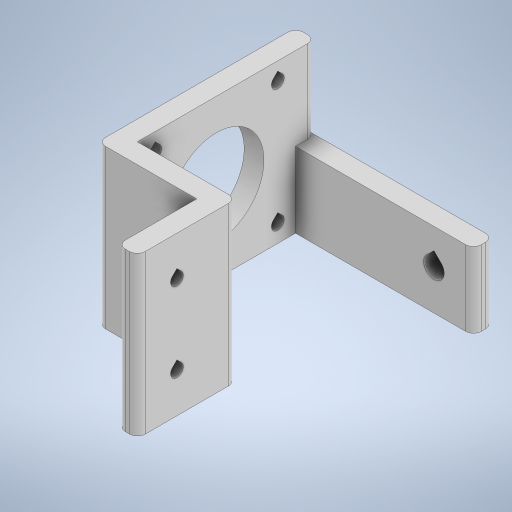
# Autodesk Inventor part: Motor Mount Redesign
Saved by Autodesk Inventor 2023.1 (Build 271208000, 208)
## iProperties
Created: 2022-11-21
Part Number: Motor Mount Redesign
Material: Generic
Document SubType Name: Modeling
Designer: nicol
Density: 1 g/cm^3
Appearance: Default
Author: nicol
Autodesk Inventor part; units mm, degrees
ref_plane "YZ Plane" through (0, 0, 0) normal (1, 0, 0) x (0, 1, 0)
ref_plane "XZ Plane" through (0, 0, 0) normal (0, 1, 0) x (-1, 0, 0)
ref_plane "XY Plane" through (0, 0, 0) normal (0, 0, 1) x (1, 0, 0)
sketch "Sketch1" plane through (0, 0, 0) normal (0, 1, 0) x (-1, 0, 0)
  line L0 (0, 0) -> (0, -25)
  line L1 (0, -25) -> (25, -25)
  line L2 (25, -25) -> (25, -65)
  line L3 (25, -65) -> (-20, -65)
  line L4 (-20, -65) -> (-20, -70)
  line L5 (-20, -70) -> (30, -70)
  line L6 (30, -70) -> (30, -20)
  line L7 (30, -20) -> (5, -20)
  line L8 (5, -20) -> (5, 0)
  line L9 (5, 0) -> (0, 0)
  line L10 (25, -65) -> (25, -70)
  dimension "d0" = 5
  dimension "d1" = 5
  dimension "d2" = 5
  dimension "d3" = 5
  dimension "d4" = 50
  dimension "d5" = 20
  dimension "d6" = 30
  dimension "d25" = 50
  constraints: 22 end point, 8 perpendicular, 2 vertical, 1 point on line
  measures "d0" distance between parallel lines of L5 L3
  measures "d1" distance between parallel lines of L6 L2
  measures "d2" distance between parallel lines of L7 L1
  measures "d3" distance between parallel lines of L8 L0
  measures "d4" distance of L5.end L6.end
  measures "d5" distance from line of L8.end L7
  measures "d6" distance between parallel lines of L0 L6
  measures "d25" distance of L4.end L5.end
extrude "Extrusion1" add sketch "Sketch1" along normal blind 40 contours L9 L8 L7 L6 L5 L10 L2 L1 L0
extrude "Extrusion2" add sketch "Sketch1" along normal blind 19 contours L10 L5 L4 L3
sketch "Sketch2" plane through (-25, 0, -25) normal (1, 0, 0) x (0, 0, -1)
  line L0 (4.5, 35.5) -> (35.5, 35.5) construction
  line L1 (35.5, 35.5) -> (35.5, 4.5) construction
  line L2 (35.5, 4.5) -> (4.5, 4.5) construction
  line L3 (4.5, 4.5) -> (4.5, 35.5) construction
  line L4 (0, 0) -> (40, 0) construction
  line L5 (0, 40) -> (45, 40) construction
  line L6 (0, 0) -> (0, 40) construction
  line L7 (0, 0) -> (0, 40) construction
  line L8 (45, 19) -> (45, 40) projected
  line L9 (40, 0) -> (40, 19) projected
  line L10 (40, 19) -> (45, 19) projected
  point P0 (-25, 0)
  point P1 (4.5, 20)
  point P2 (0, 20)
  point P3 (20, 35.5)
  point P4 (22.5, 40)
  point P5 (20, 20)
  point P6 (20, 0)
  point P7 (20, 4.5)
  dimension "d9" = 31
  dimension "d10" = 31
  constraints: 8 end point, 6 midpoint, 4 coincident, 2 horizontal alignment, 2 parallel, 2 vertical alignment, 1 horizontal, 1 perpendicular
  measures "d9" distance of L1.end L2.end
  measures "d10" distance of L0.end L1.end
hole "Hole1" at (-25, 35.5, -29.5) at (-25, 35.5, -60.5) at (-25, 4.5, -60.5) at (-25, 4.5, -29.5) direction (-1, 0, 0) diameter 3.2 depth 25.4 tip angle 118
hole "Hole2" at (-25, 20, -45) direction (-1, 0, 0) diameter 24 depth 25.4 tip angle 118
sketch "Sketch3" plane through (-5, 0, -20) normal (-1, 0, 0) x (0, 0, 1)
  line L0 (0, 40) -> (20, 40) projected
  line L1 (0, 0) -> (20, 0) projected
  point P0 (10, 30)
  point P1 (10, 10)
  point P2 (10, 40)
  dimension "d28" = 10
  dimension "d29" = 10
  constraints: 2 vertical alignment, 1 midpoint
  measures "d28" distance from line of L1 point (10, 10)
  measures "d29" distance from line of L0 point (10, 30)
hole "Hole3" at (-5, 30, -10) at (-5, 10, -10) direction (1, 0, 0) diameter 3.2 depth 25.4 tip angle 118
sketch "Sketch4" plane through (-25, 40, -70) normal (0, 0, -1) x (-1, 0, 0)
  line L0 (-45, -40) -> (5, -40) projected
  line L1 (-45, -40) -> (-45, -21) projected
  point P0 (-25, -40)
  point P1 (-35, -30)
  dimension "d37" = 10
  dimension "d38" = 10
  measures "d37" distance from line of L0 point (-35, -30)
  measures "d38" distance from line of L1 point (-35, -30)
hole "Hole4" at (10, 10, -70) direction (0, 0, 1) diameter 5.2 depth 25.4 tip angle 118
fillet "Fillet1" radius 2 8 edges at (-25, 29.5, -70) (-30, 20, -70) (-30, 20, -20) (0, 20, 0) (-5, 20, 0) (20, 9.5, -70) (20, 9.5, -65) (0, 20, -25)
sketch "Sketch5" plane through (-30, 0, -68) normal (-1, 0, 0) x (0, 0, 1)
  circle A0 centre (23, 20) radius 12 projected
  circle A1 centre (7.5, 4.5) radius 1.6 projected
  circle A2 centre (38.5, 35.5) radius 1.6 projected
  circle A3 centre (7.5, 35.5) radius 1.6 projected
  circle A4 centre (38.5, 4.5) radius 1.6 projected
  line L0 (46, 40) -> (46, 0) projected
  line L1 (0, 40) -> (46, 40) projected
  line L2 (0, 0) -> (0, 40) projected
  line L3 (0, 0) -> (46, 0) projected
  line L4 (66, 40) -> (66, 0) projected
  line L5 (48, 40) -> (66, 40) projected
  line L6 (48, 0) -> (48, 40) projected
  line L7 (48, 0) -> (66, 0) projected
  circle A5 centre (58, 30) radius 1.6 projected
  circle A6 centre (58, 10) radius 1.6 projected
  line L8 (7.5, 33.2373) -> (5.2373, 35.5)
  line L9 (5.2373, 35.5) -> (7.5, 37.7627)
  line L10 (7.5, 37.7627) -> (9.7627, 35.5)
  line L11 (9.7627, 35.5) -> (7.5, 33.2373)
  circle A7 centre (7.5, 35.5) radius 1.6 projected
  line L12 (7.5, 33.2373) -> (7.5, 37.7627) construction
  line L13 (5.2373, 35.5) -> (9.7627, 35.5) construction
  line L14 (38.5, 33.2373) -> (40.7627, 35.5)
  line L15 (40.7627, 35.5) -> (38.5, 37.7627)
  line L16 (38.5, 37.7627) -> (36.2373, 35.5)
  line L17 (36.2373, 35.5) -> (38.5, 33.2373)
  line L18 (38.5, 33.2373) -> (38.5, 37.7627) construction
  line L19 (40.7627, 35.5) -> (36.2373, 35.5) construction
  line L20 (58, 27.7373) -> (60.2627, 30)
  line L21 (60.2627, 30) -> (58, 32.2627)
  line L22 (58, 32.2627) -> (55.7373, 30)
  line L23 (55.7373, 30) -> (58, 27.7373)
  line L24 (58, 27.7373) -> (58, 32.2627) construction
  line L25 (60.2627, 30) -> (55.7373, 30) construction
  line L26 (58, 7.7373) -> (60.2627, 10)
  line L27 (60.2627, 10) -> (58, 12.2627)
  line L28 (58, 12.2627) -> (55.7373, 10)
  line L29 (55.7373, 10) -> (58, 7.7373)
  line L30 (58, 7.7373) -> (58, 12.2627) construction
  line L31 (60.2627, 10) -> (55.7373, 10) construction
  line L32 (38.5, 2.2373) -> (40.7627, 4.5)
  line L33 (40.7627, 4.5) -> (38.5, 6.7627)
  line L34 (38.5, 6.7627) -> (36.2373, 4.5)
  line L35 (36.2373, 4.5) -> (38.5, 2.2373)
  line L36 (38.5, 2.2373) -> (38.5, 6.7627) construction
  line L37 (40.7627, 4.5) -> (36.2373, 4.5) construction
  line L38 (7.5, 2.2373) -> (9.7627, 4.5)
  line L39 (9.7627, 4.5) -> (7.5, 6.7627)
  line L40 (7.5, 6.7627) -> (5.2373, 4.5)
  line L41 (5.2373, 4.5) -> (7.5, 2.2373)
  line L42 (7.5, 2.2373) -> (7.5, 6.7627) construction
  line L43 (9.7627, 4.5) -> (5.2373, 4.5) construction
  line L44 (23, 3.0294) -> (39.9706, 20)
  line L45 (39.9706, 20) -> (23, 36.9706)
  line L46 (23, 36.9706) -> (6.0294, 20)
  line L47 (6.0294, 20) -> (23, 3.0294)
  line L48 (23, 3.0294) -> (23, 36.9706) construction
  line L49 (39.9706, 20) -> (6.0294, 20) construction
  circle A8 centre (23, 20) radius 12 projected
  circle A9 centre (7.5, 35.5) radius 1.6 projected
  circle A10 centre (38.5, 4.5) radius 1.6 projected
  circle A11 centre (7.5, 4.5) radius 1.6 projected
  point P0 (68, 0)
  point P1 (56.8686, 11.1314)
  point P2 (59.1314, 11.1314)
  point P3 (56.8686, 31.1314)
  point P4 (59.1314, 31.1314)
  point P5 (6.3686, 5.6314)
  point P6 (8.6314, 5.6314)
  point P7 (37.3686, 5.6314)
  point P8 (39.6314, 5.6314)
  point P9 (37.3686, 36.6314)
  point P10 (39.6314, 36.6314)
  point P11 (8.6314, 36.6314)
  point P12 (6.3686, 36.6314)
  constraints: 84 end point, 14 midpoint, 14 parallel, 14 tangent, 7 perpendicular, 6 vertical, 1 horizontal
extrude "Extrusion3" cut sketch "Sketch5" against normal through all contours A1 L40 L39 | A2 L16 L15 | A3 L9 L10 | A4 L34 L33 | A5 L22 L21 | A6 L28 L27
sketch "Sketch6" plane through (18, 0, -70) normal (0, 0, -1) x (-1, 0, 0)
  circle A0 centre (8, 10) radius 2.6 projected
  line L0 (8, 6.323) -> (11.677, 10)
  line L1 (11.677, 10) -> (8, 13.677)
  line L2 (8, 13.677) -> (4.323, 10)
  line L3 (4.323, 10) -> (8, 6.323)
  line L4 (8, 6.323) -> (8, 13.677) construction
  line L5 (11.677, 10) -> (4.323, 10) construction
  point P0 (18, 0)
  point P1 (6.1615, 11.8385)
  point P2 (9.8385, 11.8385)
  constraints: 12 end point, 2 midpoint, 2 parallel, 2 tangent, 1 perpendicular, 1 vertical
extrude "Extrusion4" cut sketch "Sketch6" against normal blind 10 contours A0 L2 L1
equation "\"d38\" = d37"
body "Solid1"
